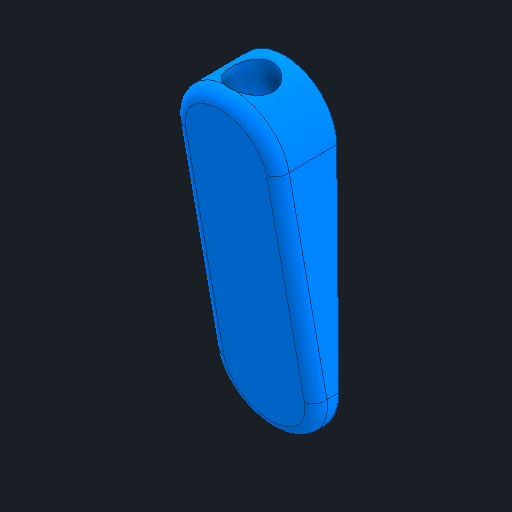
# Autodesk Inventor part: shaft_outlet
Saved by Autodesk Inventor 2023 (Build 270158030, 158C)
## iProperties
Created: 2022-03-28
Part Number: shaft_outlet
Material: Generic
Document SubType Name: Modeling
Designer: kardo
Density: 1 g/cm^3
Appearance: Blue Plastic
Mass: 2.52542 g
Surface Area: 18.6998 cm^2
Volume: 2.52542 cm^3
Author: kardo
Autodesk Inventor part; units mm, degrees
ref_plane "YZ Plane" through (0, 0, 0) normal (1, 0, 0) x (0, 1, 0)
ref_plane "XZ Plane" through (0, 0, 0) normal (0, 1, 0) x (-1, 0, 0)
ref_plane "XY Plane" through (0, 0, 0) normal (0, 0, 1) x (1, 0, 0)
derived "stencil_frame.ipt"
sketch "sk_drivetrain_profile" plane through (6, 0, 0) normal (1, 0, 0) x (0, 1, 0)
  line L0 (-529.1844, 0) -> (410.1064, 0) construction
  line L1 (-345, 3089.1136) -> (-345, -1866.0023) construction
  line L2 (0, 3089.1136) -> (0, -1866.0023) construction
  line L3 (-133.502, 53.1159) -> (-126.9655, 25.8896)
  line L4 (-377, 0) -> (-313.1973, 5.0214)
  line L5 (-130.2338, 39.5028) -> (-226.4223, 16.4099)
  line L6 (-283.6394, 7.3476) -> (-254.6742, 9.6272) construction
  line L7 (-254.6742, 9.6272) -> (-226.4223, 16.4099) construction
  line L8 (-126.9655, 25.8896) -> (-126.9655, 20.8896) construction
  line L9 (-313.1973, 5.0214) -> (-283.6394, 7.3476)
  line L10 (-844.2225, 3013.4797) -> (331.7536, -1884.8132) construction
  spline S0 degree 2 poles (-283.6394, 7.3476) (-254.6742, 9.6272) (-226.4223, 16.4099) knots 1 1 1 2 2 2
  line L11 (-227.0708, 19.1113) -> (-130.8823, 42.2041) construction
  line L12 (-129.5852, 36.8014) -> (-225.7737, 13.7086) construction
  line L13 (-227.0708, 19.1113) -> (-225.7737, 13.7086) construction
  line L14 (0, 21.3303) -> (-241.5001, 18.9703) construction
  line L15 (-48.9013, 21.6524) -> (-303.0379, 19.169) construction
  point P0 (0, 0)
  point P1 (-214.6653, 19.2325)
  point P2 (-202.2599, 19.3538)
  point P3 (-198.7861, 20.1877)
sketch "sk_prop_shaft_cut" plane through (6, 0, 21.3303) normal (0, -0.0097716, 0.9999523) x (0, -0.9999523, -0.0097716)
  line L0 (227.0817, -4.7781) -> (198.7877, -4.7781)
  line L1 (227.0817, 4.7781) -> (198.7877, 4.7781)
  arc A0 (198.7877, 4.7781) -> (198.7877, -4.7781) centre (198.7877, 0) ccw
  arc A1 (227.0817, -4.7781) -> (227.0817, 4.7781) centre (227.0817, 0) ccw
  point P0 (0.2084, -6)
  point P1 (214.6756, 0)
  point P2 (202.2695, 0)
ref_plane "plane_motor_mount" through (0, -120.75, 0) normal (0, 0.9723699, 0.2334454) x (-1, 0, 0)
derived "parameters_powertrain.ipt"
derived "parameters_frame.ipt"
extrude "lower_plate" add sketch "sk_prop_shaft_cut" along normal blind 0.8
sketch "sk_upper_plate" plane through (6, -227.0786, 19.9113) normal (0, -0.0097716, 0.9999523) x (1, 0, 0)
  line L0 (-4.7781, 28.2939) -> (-4.7781, 0) projected
  arc A0 (-4.7781, 0) -> (4.7781, 0) centre (0, 0) ccw projected
  line L1 (4.7781, 0) -> (4.7781, 28.2939) projected
  arc A1 (4.7781, 28.2939) -> (-4.7781, 28.2939) centre (0, 28.2939) ccw projected
  line L2 (-6.7781, 0) -> (-6.7781, 28.2939)
  arc A2 (6.7781, 28.2939) -> (-6.7781, 28.2939) centre (0, 28.2939) ccw
  line L3 (6.7781, 28.2939) -> (6.7781, 0)
  arc A3 (-6.7781, 0) -> (6.7781, 0) centre (0, 0) ccw
  point P0 (-6, 226.8732)
  dimension "d6" = 2
  constraints: 4 end point, 4 point on circle, 2 centre point, 3 other
  measures "d6" distance between parallel lines of L2 L0
extrude "upper_plate" add sketch "sk_upper_plate" along normal blind 8.89 contours A1 L1 A0 L0 | L2 A2 L3 A3
sketch "sk_trim" plane through (12.7781, -227.0786, 19.9113) normal (1, 0, 0) x (0, 0.0097716, -0.9999523)
  line L0 (-1.9447, -6.7781) -> (-8.89, 35.0721)
  line L1 (0, 0) -> (0, -6.7781) projected
  line L2 (-8.89, 35.0721) -> (-8.89, 28.2939) projected
  line L3 (0, -6.7781) -> (-1.9447, -6.7781)
  line L4 (-1.9447, -6.7781) -> (-8.89, -6.7781)
  line L5 (-8.89, -6.7781) -> (-8.89, 28.2939)
  dimension "d16" = 1.9447
  constraints: 8 end point, 2 collinear, 1 perpendicular
  measures "d16" distance of L1.end L0.start
extrude "trim" cut sketch "sk_trim" against normal through all
sketch "sk_drill" plane through (0, -120.75, 0) normal (0, 0.9723699, 0.2334454) x (-1, 0, 0)
  circle A0 centre (-6, 40.6252) radius 2.7781
  point P0 (0, -28.1885)
  dimension "d9" = 5.5563
  constraints: 1 centre point, 1 coincident
  measures "d9" diameter of A0
extrude "drill" cut sketch "sk_drill" along normal through all both and the other way through all
fillet "Fillet1" radius 1.5 6 edges at (10.7929, -231.8935, 22.1385) (1.2071, -231.8935, 22.1385) (-0.7781, -212.9853, 25.4666) (10.7929, -194.0771, 28.7947) (1.2071, -194.0771, 28.7947) (12.7781, -212.9853, 25.4666)
equation "\"d4\" = shell_thickness"
equation "\"d7\" = 1.6 * prop_shaft_sleeve_od"
equation "\"d16\" = 0.35 * prop_shaft_sleeve_od"
equation "\"d9\" = prop_shaft_sleeve_od"
equation "\"shell_thickness\" = 0.8"
equation "\"prop_shaft_sleeve_od\" = 5.55625"
body "Solid1"
